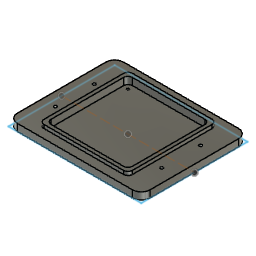
0728_base_plate (Autodesk Fusion 360 design; units mm, degrees)
Autodesk Fusion 360 part; units mm, degrees
sketch "스케치1" plane through (0, 0, 0) normal (0, 0, 1) x (1, 0, 0)
  line L0 (-63.1023, 51.7762) -> (86.8977, 51.7762)
  line L1 (86.8977, 51.7762) -> (86.8977, -68.2238)
  line L2 (86.8977, -68.2238) -> (-63.1023, -68.2238)
  line L3 (-63.1023, -68.2238) -> (-63.1023, 51.7762)
  line L4 (-63.1023, -8.2238) -> (86.8977, -8.2238) construction
  point P0 (-63.1023, -8.2238)
  point P1 (86.8977, -8.2238)
  point P2 (11.8977, -8.2238)
  dimension "d1" = 150
  dimension "d2" = 120
  constraint horizontal L0
  constraint vertical L1
  constraint horizontal L2
  constraint vertical L3
  constraint midpoint L3 P0
  constraint midpoint L1 P1
  constraint coincident P0 L4.start
  constraint coincident P1 L4.end
  constraint midpoint L4 P2
  measures "d1" distance of L0.start L0.end
  measures "d2" distance of L0.start L2.end
sketch "스케치3" plane through (0, 0, 0) normal (0, 0, 1) x (1, 0, 0)
extrude "돌출2" add sketch "스케치1" along normal blind 8
sketch "스케치4" plane through (0, 0, 8) normal (0, 0, 1) x (-1, 0, 0)
  line L0 (63.1023, 68.2238) -> (-86.8977, 68.2238)
  line L1 (-86.8977, 68.2238) -> (-86.8977, -51.7762)
  line L2 (-86.8977, -51.7762) -> (63.1023, -51.7762)
  line L3 (63.1023, -51.7762) -> (63.1023, 68.2238)
  line L4 (38.1023, -41.7762) -> (-61.8977, -41.7762)
  line L5 (-61.8977, -41.7762) -> (-61.8977, 58.2238)
  line L6 (-61.8977, 58.2238) -> (38.1023, 58.2238)
  line L7 (38.1023, 58.2238) -> (38.1023, -41.7762)
  line L8 (34.1023, -37.7762) -> (-57.8977, -37.7762)
  line L9 (-57.8977, -37.7762) -> (-57.8977, 54.2238)
  line L10 (-57.8977, 54.2238) -> (34.1023, 54.2238)
  line L11 (34.1023, 54.2238) -> (34.1023, -37.7762)
  line L12 (63.1023, -51.7762) -> (-86.8977, -51.7762)
  line L13 (-86.8977, 68.2238) -> (63.1023, 68.2238)
  line L14 (-11.8977, -51.7762) -> (-11.8977, 68.2238) construction
  line L15 (63.1023, 68.2238) -> (63.1023, -51.7762) construction
  line L16 (63.1023, 8.2238) -> (-86.8977, 8.2238) construction
  line L17 (-11.8977, -41.7762) -> (-11.8977, 58.2238) construction
  line L18 (38.1023, 8.2238) -> (-61.8977, 8.2238) construction
  line L19 (34.1023, 8.2238) -> (-57.8977, 8.2238) construction
  point P0 (-11.8977, -51.7762)
  point P1 (-11.8977, 68.2238)
  point P2 (63.1023, 8.2238)
  point P3 (-86.8977, 8.2238)
  point P4 (-11.8977, -41.7762)
  point P5 (-11.8977, 58.2238)
  point P6 (38.1023, 8.2238)
  point P7 (-61.8977, 8.2238)
  point P8 (-11.8977, 8.2238)
  point P9 (34.1023, 8.2238)
  point P10 (-57.8977, 8.2238)
  point P11 (-11.8977, 8.2238)
  point P12 (-11.8977, 8.2238)
  dimension "d9" = 100
  dimension "d10" = 100
  dimension "d11" = 92
  dimension "d12" = 92
  constraint horizontal L4
  constraint vertical L5
  constraint horizontal L6
  constraint vertical L7
  constraint horizontal L8
  constraint vertical L9
  constraint horizontal L10
  constraint vertical L11
  constraint coincident L2 P0
  constraint coincident L0 P1
  constraint midpoint P0 L12
  constraint midpoint P1 L13
  constraint coincident P0 L14.start
  constraint coincident P1 L14.end
  constraint coincident L3 P2
  constraint midpoint L1 P3
  constraint midpoint P2 L15
  constraint coincident P2 L16.start
  constraint coincident P3 L16.end
  constraint midpoint L4 P4
  constraint midpoint L6 P5
  constraint midpoint L7 P6
  constraint midpoint L5 P7
  constraint coincident P4 L17.start
  constraint coincident P5 L17.end
  constraint coincident P6 L18.start
  constraint coincident P7 L18.end
  constraint midpoint L17 P12
  constraint midpoint L11 P9
  constraint midpoint L9 P10
  constraint coincident P9 L19.start
  constraint coincident P10 L19.end
  constraint midpoint L19 P12
  constraint midpoint L14 P12
  constraint coincident P12 P11
  measures "d9" distance of L4.start L4.end
  measures "d10" distance of L4.start L6.end
  measures "d11" distance of L8.start L8.end
  measures "d12" distance of L8.start L10.end
extrude "돌출3" add sketch "스케치4" along normal blind 4 contours L4 L5 L6 L7
extrude "돌출4" cut 1 faces at (-3.4356, 7.1096, 8) along direction (0, 0, -1) blind 4
sketch "스케치6" plane through (0, 0, 0) normal (0, 0, 1) x (1, 0, 0)
sketch "스케치7" plane through (0, 0, 0) normal (0, 0, 1) x (1, 0, 0)
  line L0 (71.8977, 13.7762) -> (-48.1023, 13.7762) construction
  line L1 (-48.1023, 13.7762) -> (-48.1023, -30.2238) construction
  line L2 (-48.1023, -30.2238) -> (71.8977, -30.2238) construction
  line L3 (71.8977, -30.2238) -> (71.8977, 13.7762) construction
  line L4 (71.8977, -8.2238) -> (-48.1023, -8.2238) construction
  circle A0 centre (71.8977, 13.7762) radius 2
  circle A1 centre (71.8977, -30.2238) radius 2
  circle A2 centre (-48.1023, 13.7762) radius 2
  circle A3 centre (-48.1023, -30.2238) radius 2
  point P0 (71.8977, -8.2238)
  point P1 (-48.1023, -8.2238)
  point P2 (11.8977, -8.2238)
  point P3 (11.8977, -8.2238)
  dimension "d17" = 120
  dimension "d18" = 44
  dimension "d19" = 4
  dimension "d20" = 4
  constraint horizontal L0
  constraint vertical L1
  constraint horizontal L2
  constraint vertical L3
  constraint midpoint L3 P0
  constraint midpoint L1 P1
  constraint coincident P0 L4.start
  constraint coincident P1 L4.end
  constraint midpoint L4 P3
  constraint coincident P3 P2
  constraint coincident L0.start L3.end
  constraint coincident L2.end L3.start
  constraint coincident L0.end L1.start
  constraint coincident L1.end L2.start
  constraint equal A0 A2
  constraint equal A1 A3
  measures "d17" distance of L0.start L0.end
  measures "d18" distance of L0.start L2.end
  measures "d19" diameter of A0
  measures "d20" diameter of A1
extrude "돌출5" cut sketch "스케치7" along normal blind 10
sketch "스케치8" plane through (0, 0, 4) normal (0, 0, 1) x (-1, 0, 0)
  line L0 (-57.8977, 54.2238) -> (-57.8977, -37.7762)
  line L1 (-57.8977, -37.7762) -> (34.1023, -37.7762)
  line L2 (34.1023, -37.7762) -> (34.1023, 54.2238)
  line L3 (34.1023, 54.2238) -> (-57.8977, 54.2238)
  line L4 (28.1023, -31.7762) -> (-51.8977, -31.7762) construction
  line L5 (-51.8977, -31.7762) -> (-51.8977, 48.2238) construction
  line L6 (-51.8977, 48.2238) -> (28.1023, 48.2238) construction
  line L7 (28.1023, 48.2238) -> (28.1023, -31.7762) construction
  line L8 (34.1023, 8.2238) -> (-57.8977, 8.2238) construction
  line L9 (28.1023, 8.2238) -> (-51.8977, 8.2238) construction
  circle A0 centre (28.1023, -31.7762) radius 3.5748
  circle A1 centre (-51.8977, -31.7762) radius 3.0869
  circle A2 centre (-51.8977, 48.2238) radius 2.1374
  circle A3 centre (28.1023, 48.2238) radius 4.474
  point P0 (34.1023, 8.2238)
  point P1 (-57.8977, 8.2238)
  point P2 (-11.8977, 8.2238)
  point P3 (28.1023, 8.2238)
  point P4 (-51.8977, 8.2238)
  point P5 (-11.8977, 8.2238)
  dimension "d23" = 80
  dimension "d24" = 80
  constraint horizontal L4
  constraint vertical L5
  constraint horizontal L6
  constraint vertical L7
  constraint midpoint L2 P0
  constraint midpoint L0 P1
  constraint coincident P0 L8.start
  constraint coincident P1 L8.end
  constraint midpoint L8 P5
  constraint midpoint L7 P3
  constraint midpoint L5 P4
  constraint coincident P3 L9.start
  constraint coincident P4 L9.end
  constraint midpoint L9 P5
  constraint coincident P5 P2
  constraint coincident L4.start L7.end
  constraint coincident L4.end L5.start
  constraint coincident L5.end L6.start
  constraint coincident L6.end L7.start
  measures "d23" distance of L4.start L4.end
  measures "d24" distance of L4.start L6.end
extrude "돌출6" cut sketch "스케치8" against normal blind 5 contours A0 | A1 | A2 | A3
fillet "모깎기6" radius 10 1 edges at (86.8977, -68.2238, 4)
fillet "모깎기7" radius 10 1 edges at (86.8977, 51.7762, 4)
fillet "모깎기8" radius 5 1 edges at (61.8977, -58.2238, 10)
fillet "모깎기9" radius 5 1 edges at (61.8977, 41.7762, 10)
fillet "모깎기10" radius 5 1 edges at (-38.1023, -58.2238, 10)
fillet "모깎기11" radius 5 1 edges at (-38.1023, 41.7762, 10)
fillet "모깎기12" radius 10 1 edges at (-63.1023, -68.2238, 4)
fillet "모깎기13" radius 10 1 edges at (-63.1023, 51.7762, 4)
fillet "모깎기14" radius 5 1 edges at (57.8977, -54.2238, 8)
fillet "모깎기15" radius 5 1 edges at (57.8977, 37.7762, 8)
fillet "모깎기16" radius 5 1 edges at (-34.1023, 37.7762, 8)
fillet "모깎기17" radius 5 1 edges at (-34.1023, -54.2238, 8)
thread "스레드1" "ISO Metric profile 3.0 M3x0.5 6H" major diameter 3.086 minor diameter 2.529 pitch 0.5 angle 60 resizes the face on face at (-31.6593, 32.1322, 1.3333)
thread "스레드2" "ISO Metric profile 3.0 M3x0.5 6H" major diameter 3.086 minor diameter 2.529 pitch 0.5 angle 60 resizes the face on face at (-32.5541, -47.7783, 1.3333)
thread "스레드3" "ISO Metric profile 3.0 M3x0.5 6H" major diameter 3.086 minor diameter 2.529 pitch 0.5 angle 60 resizes the face on face at (48.8262, 32.0836, 1.3333)
thread "스레드4" "ISO Metric profile 3.0 M3x0.5 6H" major diameter 3.086 minor diameter 2.529 pitch 0.5 angle 60 resizes the face on face at (49.7709, -48.011, 1.3333)
thread "스레드5" "ISO Metric profile 4.0 M4x0.7 6H" major diameter 4.1095 minor diameter 3.332 pitch 0.7 angle 60 resizes the face on face at (73.492, 14.9838, 2.6667)
thread "스레드6" "ISO Metric profile 4.0 M4x0.7 6H" major diameter 4.1095 minor diameter 3.332 pitch 0.7 angle 60 resizes the face on face at (70.5012, -31.6555, 5.3333)
thread "스레드7" "ISO Metric profile 4.0 M4x0.7 6H" major diameter 4.1095 minor diameter 3.332 pitch 0.7 angle 60 resizes the face on face at (-46.1048, 13.8759, 2.6667)
thread "스레드8" "ISO Metric profile 4.0 M4x0.7 6H" major diameter 4.1095 minor diameter 3.332 pitch 0.7 angle 60 resizes the face on face at (-46.1048, -30.1241, 2.6667)
fillet "모깎기1" [suppressed]
fillet "모깎기2" [suppressed]
fillet "모깎기3" [suppressed]
fillet "모깎기4" [suppressed]
fillet "모깎기5" [suppressed]
sketch "스케치5" plane through (0, 0, 8) normal (0, 0, 1) x (-1, 0, 0)
  line L0 (63.1023, 68.2238) -> (-86.8977, 68.2238)
  line L1 (-86.8977, 68.2238) -> (-86.8977, -51.7762)
  line L2 (-86.8977, -51.7762) -> (63.1023, -51.7762)
  line L3 (63.1023, -51.7762) -> (63.1023, 68.2238)
  line L4 (38.1023, 58.2238) -> (38.1023, -41.7762)
  line L5 (38.1023, -41.7762) -> (-61.8977, -41.7762)
  line L6 (-61.8977, -41.7762) -> (-61.8977, 58.2238)
  line L7 (-61.8977, 58.2238) -> (38.1023, 58.2238)
  line L8 (52.6316, -44.9948) -> (-78.4313, -44.9948) construction
  line L9 (-78.4313, -44.9948) -> (-78.4313, 47.678) construction
  line L10 (-78.4313, 47.678) -> (52.6316, 47.678) construction
  line L11 (52.6316, 47.678) -> (52.6316, -44.9948) construction
  constraint horizontal L8
  constraint vertical L9
  constraint horizontal L10
  constraint vertical L11
extrude "돌출1" [suppressed]
sketch "스케치2" plane through (0, 0, 8) normal (0, 0, 1) x (-1, 0, 0)
  line L0 (63.1023, 48.2238) -> (-86.8977, 48.2238)
  line L1 (-86.8977, 48.2238) -> (-86.8977, -51.7762)
  line L2 (-86.8977, -51.7762) -> (63.1023, -51.7762)
  line L3 (63.1023, -51.7762) -> (63.1023, 48.2238)
  line L4 (40.9967, -38.1097) -> (-57.0033, -38.1097)
  line L5 (-57.0033, -38.1097) -> (-57.0033, 32.143)
  line L6 (-57.0033, 32.143) -> (40.9967, 32.143)
  line L7 (40.9967, 32.143) -> (40.9967, -38.1097)
  line L8 (26.9462, -28.1011) -> (-55, -28.1011)
  line L9 (-55, -28.1011) -> (-55, 20)
  line L10 (-55, 20) -> (26.9462, 20)
  line L11 (26.9462, 20) -> (26.9462, -28.1011)
  dimension "d5" = 98
  dimension "d6" = 70.2526
  constraint horizontal L4
  constraint vertical L5
  constraint horizontal L6
  constraint vertical L7
  constraint horizontal L8
  constraint vertical L9
  constraint horizontal L10
  constraint vertical L11
  measures "d5" distance of L4.start L4.end
  measures "d6" distance of L4.start L6.end
